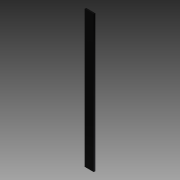
# Autodesk Inventor part: plaskownik_30x5mm_45cm
Saved by Autodesk Inventor 2015 (Build 190159000, 159)
## iProperties
Created: 2017-05-03
Part Number: plaskownik_30x5mm_45cm
Material: Generic
Document SubType Name: Modeling
Designer: miki
Density: 1 g/cm^3
Appearance: Glossy - Black
Author: miki
Autodesk Inventor part; units mm, degrees
ref_plane "YZ Plane" through (0, 0, 0) normal (1, 0, 0) x (0, 1, 0)
ref_plane "XZ Plane" through (0, 0, 0) normal (0, 1, 0) x (-1, 0, 0)
ref_plane "XY Plane" through (0, 0, 0) normal (0, 0, 1) x (1, 0, 0)
sketch "Sketch1" plane through (0, 0, 0) normal (0, 0, 1) x (1, 0, 0)
  line L0 (0, 0) -> (30, 0)
  line L1 (30, 0) -> (30, -5)
  line L2 (30, -5) -> (0, -5)
  line L3 (0, -5) -> (0, 0)
  dimension "d0" = 30
  dimension "d1" = 5
  constraints: 8 end point, 2 parallel, 1 horizontal, 1 perpendicular
  measures "d0" distance of L1.end L2.end
  measures "d1" distance of L0.end L1.end
extrude "Extrusion1" add sketch "Sketch1" along normal blind 450
body "Solid1"
